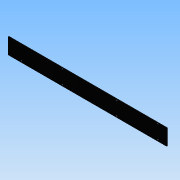
# Autodesk Inventor part: electronics
Saved by Autodesk Inventor 2015 (Build 190159000, 159)
## iProperties
Created: 2016-04-17
Part Number: electronics
Material: Générique
Document SubType Name: Modeling
Designer: Gregwar
Density: 1 g/cm^3
Appearance: Par défaut
Author: Gregwar
Autodesk Inventor part; units mm, degrees
ref_plane "YZ Plane" through (0, 0, 0) normal (1, 0, 0) x (0, 1, 0)
ref_plane "XZ Plane" through (0, 0, 0) normal (0, 1, 0) x (-1, 0, 0)
ref_plane "XY Plane" through (0, 0, 0) normal (0, 0, 1) x (1, 0, 0)
sketch "Esquisse1" plane through (0, 0, 0) normal (0, 1, 0) x (-1, 0, 0)
  line L0 (0, 0) -> (250, 0)
  line L1 (250, 0) -> (250, -25)
  line L2 (250, -25) -> (0, -25)
  line L3 (0, -25) -> (0, 0)
  line L4 (14.24, 0) -> (14.24, -25) construction
  line L5 (0, -12.5) -> (250, -12.5) construction
  circle A0 centre (14.24, -1.8) radius 1.5
  circle A1 centre (14.24, -23.2) radius 1.5
  circle A2 centre (79.24, -1.8) radius 1.5
  circle A3 centre (79.24, -23.2) radius 1.5
  line L6 (229.7, 0) -> (229.7, -25) construction
  circle A4 centre (229.7, -1.8) radius 1.5
  circle A5 centre (229.7, -23.2) radius 1.5
  circle A6 centre (165, -1.8) radius 1.5
  circle A7 centre (165, -23.2) radius 1.5
  dimension "d0" = 25
  dimension "d1" = 250
  dimension "d2" = 1.8
  dimension "d3" = 3
  dimension "d4" = 14.24
  dimension "d7" = 65
  dimension "d12" = 3
  dimension "d13" = 1.8
  dimension "d17" = 64.7
  dimension "d32" = 165
  constraints: 14 end point, 8 centre point, 6 point on line, 3 horizontal, 2 midpoint, 2 parallel, 2 perpendicular, 2 symmetric about line, 1 vertical, 10 other
  measures "d0" distance of L2.end L0.start
  measures "d1" distance of L0.start L0.end
  measures "d2" distance from line of L0 A0.centre
  measures "d3" diameter of A0
  measures "d4" distance between parallel lines of L3 L4
  measures "d7" distance of A1.centre A3.centre
  measures "d12" diameter of A4
  measures "d13" distance from line of L0 A4.centre
  measures "d17" distance of A4.centre A6.centre
  measures "d32" distance from line of L3 A7.centre
extrude "Extrusion1" add sketch "Esquisse1" along normal blind 1.6
sketch "Esquisse2" plane through (0, 1.6, 0) normal (0, 1, 0) x (1, 0, 0)
  circle A0 centre (-165, 23.2) radius 1.5 construction
  circle A1 centre (-165, 1.8) radius 1.5 construction
  circle A2 centre (-229.7, 23.2) radius 1.5 construction
  circle A3 centre (-229.7, 1.8) radius 1.5 construction
  circle A4 centre (-79.24, 1.8) radius 1.5 construction
  circle A5 centre (-79.24, 23.2) radius 1.5 construction
  circle A6 centre (-14.24, 23.2) radius 1.5 construction
  circle A7 centre (-14.24, 1.8) radius 1.5 construction
  line L0 (-250, 0) -> (0, 0) construction
  line L1 (0, 0) -> (0, 25) construction
  line L2 (0, 25) -> (-250, 25) construction
  line L3 (-250, 25) -> (-250, 0) construction
  line L4 (-250, 8) -> (-236, 8)
  line L5 (-236, 8) -> (-236, 20)
  line L6 (-236, 20) -> (-250, 20)
  line L7 (-250, 20) -> (-250, 8)
  line L8 (-250, 14) -> (-236, 14) construction
  dimension "d24" = 14
  dimension "d25" = 14
  dimension "d26" = 12
  constraints: 10 end point, 2 midpoint, 2 parallel, 1 horizontal, 1 perpendicular, 1 point on line
  measures "d24" distance between parallel lines of L0 L8
  measures "d25" distance between parallel lines of L3 L5
  measures "d26" distance between parallel lines of L6 L4
extrude "Extrusion2" add sketch "Esquisse2" along normal blind 7
sketch "Esquisse3" plane through (-250, 0, -25) normal (-1, 0, 0) x (0, 0, 1)
  line L0 (25, 0) -> (0, 0) projected
  line L1 (25, 0) -> (25, 1.6) projected
  line L2 (17, 1.6) -> (25, 1.6) projected
  line L3 (17, 1.6) -> (17, 8.6) projected
  line L4 (5, 6.6) -> (17, 6.6) projected
  line L5 (5, 1.6) -> (5, 8.6) projected
  line L6 (0, 1.6) -> (5, 1.6) projected
  line L7 (0, 0) -> (0, 1.6) projected
  line L8 (5, 8.6) -> (17, 8.6) construction
  line L9 (11, 6.6) -> (11, 0) construction
  circle A0 centre (11, 4.1) radius 1.25
  dimension "d29" = 2.5
  constraints: 2 end point, 2 point on line, 1 centre point, 1 vertical, 2 other
  measures "d29" diameter of A0
equation "\"d12\" = d3"
equation "\"d13\" = d2"
